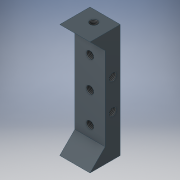
# Autodesk Inventor part: Part2
Saved by Autodesk Inventor 2017 SP1 (Build 210196100, 196)
## iProperties
Created: 2017-05-15
Part Number: Part2
Material: ABS Plastic
Document SubType Name: Modeling
Designer: zallen
Density: 1.06 g/cm^3
Appearance: CR Dark Blue
Mass: 16.1468 g
Surface Area: 68.8305 cm^2
Volume: 15.2329 cm^3
Author: zallen
Autodesk Inventor part; units mm, degrees
ref_plane "YZ Plane" through (0, 0, 0) normal (1, 0, 0) x (0, 1, 0)
ref_plane "XZ Plane" through (0, 0, 0) normal (0, 1, 0) x (-1, 0, 0)
ref_plane "XY Plane" through (0, 0, 0) normal (0, 0, 1) x (1, 0, 0)
sketch "Sketch1" plane through (0, 0, 0) normal (0, 0, 1) x (1, 0, 0)
  line L0 (-10, -27.5) -> (10, -27.5)
  line L1 (10, -27.5) -> (10, 27.5)
  line L2 (10, 27.5) -> (-10, 27.5)
  line L3 (-10, 27.5) -> (-10, -27.5)
  line L4 (-10, -27.5) -> (10, 27.5) construction
  line L5 (10, -27.5) -> (-10, 27.5) construction
  point P0 (0, 0)
  dimension "d0" = 20
  dimension "d1" = 55
  constraints: 12 end point, 2 midpoint, 2 parallel, 1 horizontal, 1 perpendicular
  measures "d0" distance of L2.end L1.end
  measures "d1" distance of L1.end L0.end
extrude "Extrusion1" add sketch "Sketch1" along normal blind 10
sketch "Sketch3" plane through (10, -27.5, 0) normal (1, 0, 0) x (0, 0, -1)
  line L0 (0, 0) -> (0, 55) construction
  line L1 (-10, 0) -> (-10, 55) projected
  line L2 (-10, 55) -> (-20, 65)
  line L3 (0, 55) -> (-10, 55)
  line L4 (-20, 65) -> (0, 65)
  line L5 (0, 65) -> (0, 55)
  line L6 (0, 27.5) -> (-50, 27.5) construction
  line L7 (-10, 0) -> (-20, -10)
  line L8 (0, 0) -> (-10, 0)
  line L9 (-20, -10) -> (0, -10)
  line L10 (0, -10) -> (0, 0)
  dimension "d8" = 20
  dimension "d12" = 10
  dimension "d13" = 50
  constraints: 18 end point, 2 symmetric about line, 1 collinear, 1 horizontal, 1 horizontal alignment
  measures "d8" distance of L2.end L4.end
  measures "d12" horizontal distance of L1.end L2.end
  measures "d13" distance of L6.start L6.end
extrude "Extrusion3" add sketch "Sketch3" against normal blind 20
sketch "Sketch4" plane through (0, 0, 10) normal (0, 0, 1) x (1, 0, 0)
  circle A0 centre (0, 20) radius 2.5
  circle A1 centre (0, 0) radius 2.5
  circle A2 centre (0, -20) radius 2.5
  dimension "d14" = 5
  dimension "d15" = 5
  dimension "d16" = 5
  dimension "d17" = 20
  dimension "d18" = 20
  constraints: 3 centre point, 1 coincident
  measures "d14" diameter of A0
  measures "d15" diameter of A1
  measures "d16" diameter of A2
  measures "d17" distance of A0.centre point (0, 0)
  measures "d18" distance of point (0, 0) A2.centre
sketch "Sketch5" plane through (10, -37.5, 0) normal (0, -1, 0) x (1, 0, 0)
  circle A0 centre (-10, 7.5) radius 2.5
  circle A1 centre (-10, 7.5) radius 2.5
  point P0 (-10, 0)
  dimension "d19" = 5
  dimension "d20" = 7.5
  dimension "d35" = 5
  constraints: 2 centre point, 1 coincident
  measures "d19" diameter of A0
  measures "d20" distance of point (-10, 0) A0.centre
  measures "d35" diameter of A1
extrude "Extrusion4" cut sketch "Sketch5" against normal blind 10
extrude "Extrusion5" cut sketch "Sketch4" against normal through all
thread "Thread1" size "M5x0.8" class "6H" standard "ANSI Metric M Profile" full length
thread "Thread2" size "M5x0.8" class "6H" standard "ANSI Metric M Profile" full length
thread "Thread3" size "M5x0.8" class "6H" standard "ANSI Metric M Profile" full length
thread "Thread4" size "M5x0.8" class "6H" standard "ANSI Metric M Profile" full length
thread "Thread5" size "M5x0.8" class "6H" standard "ANSI Metric M Profile" full length
sketch "Sketch6" plane through (10, 37.5, 20) normal (0, 1, 0) x (1, 0, 0)
  circle A0 centre (-10, 12.5) radius 2.5
  line L0 (0, 20) -> (0, 0) projected
  point P0 (-10, 20)
  dimension "d36" = 5
  dimension "d37" = 7.5
  dimension "d38" = 10
  constraints: 1 centre point
  measures "d36" diameter of A0
  measures "d37" distance of point (-10, 20) A0.centre
  measures "d38" distance from line of L0 A0.centre
extrude "Extrusion6" cut sketch "Sketch6" against normal blind 10
thread "Thread6" size "M5x0.8" class "6H" standard "ANSI Metric M Profile" full length
sketch "Sketch7" plane through (10, 37.5, 20) normal (1, 0, 0) x (0, 0, -1)
  circle A0 centre (15, -27.5) radius 2.5
  circle A1 centre (15, -47.5) radius 2.5
  line L0 (20, -35) -> (20, -40) projected
  line L1 (10, -40) -> (10, -35) projected
  line L2 (20, -75) -> (20, 0) projected
  point P0 (20, -37.5)
  dimension "d43" = 5
  dimension "d44" = 5
  dimension "d45" = 20
  dimension "d46" = 7.5
  dimension "d47" = 5
  dimension "d48" = 5
  constraints: 2 centre point
  measures "d43" diameter of A0
  measures "d44" diameter of A1
  measures "d45" distance of A1.centre A0.centre
  measures "d46" vertical distance of A0.centre L1.end
  measures "d47" distance from line of L2 A0.centre
  measures "d48" distance from line of L2 A1.centre
extrude "Extrusion7" cut sketch "Sketch7" against normal through all
thread "Thread7" size "M5x0.8" class "6H" standard "ANSI Metric M Profile" full length
thread "Thread8" size "M5x0.8" class "6H" standard "ANSI Metric M Profile" full length
body "Solid1"
